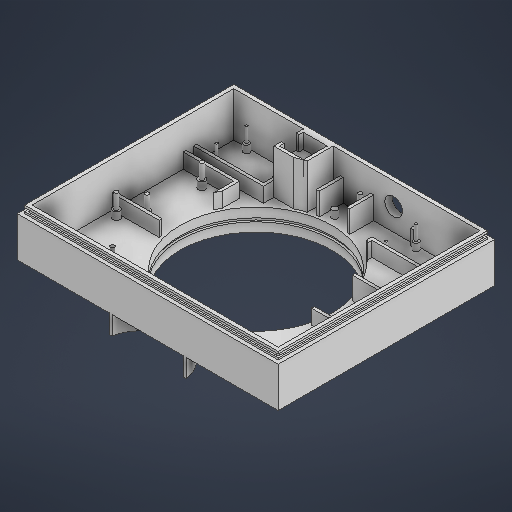
# Autodesk Inventor part: Hardware_Container-bottom-with_rods
Saved by Autodesk Inventor 2026.1 (Build 301233000, 233)
## iProperties
Created: 2025-05-15
Part Number: Hardware_Container-bottom-with_rods
Material: Générique
Document SubType Name: Modeling
Designer: ewenm
Density: 1 g/cm^3
Appearance: Par défaut
Author: ewenm
Autodesk Inventor part; units mm, degrees
ref_plane "YZ Plane" through (0, 0, 0) normal (1, 0, 0) x (0, 1, 0)
ref_plane "XZ Plane" through (0, 0, 0) normal (0, 1, 0) x (-1, 0, 0)
ref_plane "XY Plane" through (0, 0, 0) normal (0, 0, 1) x (1, 0, 0)
sketch "Esquisse1" plane through (0, 0, 0) normal (0, 1, 0) x (-1, 0, 0)
  circle A0 centre (0, 0) radius 51.25
  circle A1 centre (0, 0) radius 53.25
  dimension "d0" = 102.5
  dimension "d1" = 106.5
  constraints: 2 centre point, 2 coincident
  measures "d0" diameter of A0
  measures "d1" diameter of A1
extrude "Extrusion1" add sketch "Esquisse1" along normal blind 12.5
sketch "Esquisse5" plane through (0, 12.5, 0) normal (0, 1, 0) x (1, 0, 0)
  line L0 (-88, -73) -> (88, -73)
  line L1 (88, -73) -> (88, 73)
  line L2 (88, 73) -> (-88, 73)
  line L3 (-88, 73) -> (-88, -73)
  line L4 (-88, -73) -> (88, 73) construction
  line L5 (88, -73) -> (-88, 73) construction
  circle A0 centre (0, 0) radius 51.25
  dimension "d4" = 176
  dimension "d5" = 146
  dimension "d263" = 102.5
  constraints: 12 end point, 2 midpoint, 2 parallel, 1 centre point, 1 coincident, 1 horizontal, 1 perpendicular
  measures "d4" distance of L0.start L0.end
  measures "d5" distance of L1.end L0.end
  measures "d263" diameter of A0
extrude "Extrusion2" add sketch "Esquisse5" along normal blind 2
sketch "Esquisse8" plane through (0, 14.5, 0) normal (0, 1, 0) x (1, 0, 0)
  line L0 (88, -73) -> (88, 73)
  line L1 (88, 73) -> (-88, 73)
  line L2 (-88, 73) -> (-88, -73)
  line L3 (-88, -73) -> (88, -73)
  line L4 (88, -73) -> (-88, 73) construction
  line L5 (88, 73) -> (-88, -73) construction
  line L6 (83, -68) -> (83, 68)
  line L7 (83, 68) -> (-83, 68)
  line L8 (-83, 68) -> (-83, -68)
  line L9 (-83, -68) -> (83, -68)
  line L10 (83, -68) -> (-83, 68) construction
  line L11 (83, 68) -> (-83, -68) construction
  line L12 (88, 73) -> (-88, 73) projected
  point P0 (0, 0)
  dimension "d8" = 136
  dimension "d9" = 166
  dimension "d214" = 146
  dimension "d215" = 176
  dimension "d216" = 0
  constraints: 24 end point, 4 midpoint, 4 parallel, 2 perpendicular, 1 vertical
  measures "d8" distance of L6.start L6.end
  measures "d9" distance of L7.end L6.end
  measures "d214" distance between parallel lines of L1 L3
  measures "d215" distance between parallel lines of L2 L0
  measures "d216" distance between parallel lines of L12 L1
extrude "Extrusion3" add sketch "Esquisse8" along normal blind 25
sketch "Esquisse9" plane through (0, 39.5, 0) normal (0, 1, 0) x (1, 0, 0)
  line L0 (85.5, -70.5) -> (85.5, 70.5)
  line L1 (85.5, 70.5) -> (-85.5, 70.5)
  line L2 (-85.5, 70.5) -> (-85.5, -70.5)
  line L3 (-85.5, -70.5) -> (85.5, -70.5)
  line L4 (85.5, -70.5) -> (-85.5, 70.5) construction
  line L5 (85.5, 70.5) -> (-85.5, -70.5) construction
  line L6 (83, -68) -> (83, 68)
  line L7 (83, 68) -> (-83, 68)
  line L8 (-83, 68) -> (-83, -68)
  line L9 (-83, -68) -> (83, -68)
  line L10 (83, -68) -> (-83, 68) construction
  line L11 (83, 68) -> (-83, -68) construction
  point P0 (0, 0)
  dimension "d12" = 141
  dimension "d13" = 171
  constraints: 24 end point, 4 midpoint, 4 parallel, 2 perpendicular, 1 vertical
  measures "d12" distance of L0.start L0.end
  measures "d13" distance of L1.end L0.end
extrude "Extrusion4" add sketch "Esquisse9" along normal blind 5
sketch "Esquisse10" plane through (0, 14.5, 0) normal (0, 1, 0) x (1, 0, 0)
  line L0 (-83, -68) -> (83, -68) projected
  line L1 (-83, -68) -> (69, -68)
  line L2 (-83, -12.0588) -> (-83, -68)
  line L3 (-83, -68) -> (67, -68)
  line L4 (-83, -14.0686) -> (-83, -68)
  circle A0 centre (0, 0) radius 51.25 projected
  line L5 (69, -12) -> (49.8253, -12)
  line L6 (-49.8111, -12.0588) -> (-83, -12.0588)
  line L7 (67, -14) -> (49.3007, -14)
  line L8 (-49.2812, -14.0686) -> (-83, -14.0686)
  line L9 (67, -43) -> (69, -43)
  line L10 (67, -63) -> (69, -63)
  line L11 (67, -68) -> (67, -63)
  line L12 (67, -43) -> (67, -14)
  line L13 (69, -68) -> (69, -63)
  line L14 (69, -43) -> (69, -12)
  point P0 (51.25, 0)
  point P1 (68, -63)
  point P2 (68, -43)
  dimension "d16" = 152
  dimension "d17" = 56
  dimension "d18" = 150
  dimension "d19" = 54
  dimension "d20" = 5
  dimension "d21" = 20
  constraints: 28 end point, 8 parallel, 8 perpendicular, 5 point on circle, 2 midpoint, 2 point on line, 1 coincident
  measures "d16" distance of L0.start L1.end
  measures "d17" distance of L5.start L1.end
  measures "d18" distance of L0.start L3.end
  measures "d19" distance of L7.start L3.end
  measures "d20" distance from line of L0 point (68, -63)
  measures "d21" distance of point (68, -63) point (68, -43)
extrude "Extrusion5" add sketch "Esquisse10" along normal blind 10 contours L11 L10 L13 L0 | L6 A0 L8 L2 | A0 L5 L14 L9 L12 L7
sketch "Esquisse11" plane through (0, 14.5, 0) normal (0, 1, 0) x (1, 0, 0)
  line L0 (-83, -68) -> (-83, 68) projected
  line L1 (-83, -68) -> (67, -68) projected
  line L2 (-83, 29.4235) -> (-85.5, 61.9088)
  line L3 (-85.5, -70.5) -> (-85.5, 70.5) projected
  line L4 (-83, 33.9412) -> (-49, 33.9412)
  line L5 (-49, 33.9412) -> (-49, 15.0187)
  line L6 (-49.8111, -12.0588) -> (-83, -12.0588) projected
  line L7 (-83, 68) -> (-83, -12.0588) projected
  line L8 (-83, 35.9412) -> (-47, 35.9412)
  line L9 (-47, 35.9412) -> (-47, 20.4343)
  arc A0 (49.8253, -12) -> (-49.8111, -12.0588) centre (0, 0) ccw projected
  arc A1 (-49, 15.0187) -> (-48.1736, 17.489) centre (0, 0) ccw
  point P0 (-83, -20.5374)
  point P1 (-83, 35.9412)
  dimension "d29" = 34
  dimension "d32" = 36
  dimension "d34" = 2
  dimension "d35" = 48
  constraints: 10 end point, 5 point on circle, 5 point on line, 3 perpendicular, 1 centre point, 1 concentric, 1 horizontal
  measures "d29" distance of L4.start L4.end
  measures "d32" distance of L8.start L8.end
  measures "d34" distance between parallel lines of L4 L8
  measures "d35" distance between parallel lines of L8 L6
extrude "Extrusion6" add sketch "Esquisse11" along normal blind 10 contours L0 L8 L9 A0 L5 L4
sketch "Esquisse13" plane through (0, 14.5, 0) normal (0, 1, 0) x (1, 0, 0)
  line L0 (83, 68) -> (-83, 68) projected
  line L1 (-83, 68) -> (-83, 35.9412) projected
  line L2 (-83, 68) -> (-83, 43)
  line L3 (-83, 43) -> (-38, 43)
  line L4 (-38, 43) -> (-38, 68)
  line L5 (-38, 68) -> (-83, 68)
  line L6 (-83, 68) -> (-83, 41)
  line L7 (-83, 41) -> (-36, 41)
  line L8 (-36, 43) -> (-36, 68)
  line L9 (-36, 68) -> (-83, 68)
  line L10 (-36, 68) -> (-36, 43)
  line L11 (13.6206, 68) -> (-36, 68)
  line L12 (-36, 68) -> (-36, 41)
  line L13 (15.4407, 68) -> (-36, 68)
  circle A0 centre (0, 0) radius 51.25 projected
  line L14 (83, 68) -> (38, 68)
  line L15 (83, 43) -> (83, 68)
  line L16 (83, 68) -> (36, 68)
  line L17 (83, 41) -> (83, 68)
  point P0 (-30.4802, 41.201)
  point P1 (-27.557, 43.2108)
  dimension "d49" = 25
  dimension "d50" = 45
  dimension "d51" = 27
  dimension "d52" = 47
  constraints: 32 end point, 4 parallel, 4 point on line, 2 perpendicular, 2 point on circle, 1 collinear
  measures "d49" distance of L0.end L2.end
  measures "d50" distance of L3.end L2.end
  measures "d51" distance of L0.end L6.end
  measures "d52" distance of L7.end L6.end
extrude "Extrusion7" add sketch "Esquisse13" along normal blind 10 contours L8 L12 L7 L1 L3 L4 L0
sketch "Esquisse15" plane through (0, 14.5, 0) normal (0, 1, 0) x (1, 0, 0)
  line L0 (-83, -68) -> (-83, 68) projected
  line L1 (83, -68) -> (-83, -68) projected
  circle A0 centre (-71, -65.05) radius 1.35
  circle A1 centre (-71, -65.05) radius 2.5
  circle A2 centre (-46.9, -49.85) radius 1.35
  circle A3 centre (-46.9, -49.85) radius 2.5
  circle A4 centre (3.9, -65.05) radius 1.35
  circle A5 centre (3.9, -65.05) radius 2.5
  circle A6 centre (-77.32, -16.85) radius 1.35
  circle A7 centre (-77.32, -16.85) radius 2.5
  point P0 (0, 0)
  point P1 (-46.9, -21.95)
  dimension "d63" = 12
  dimension "d64" = 2.95
  dimension "d65" = 15.2
  dimension "d66" = 24.1
  dimension "d67" = 50.8
  dimension "d68" = 0
  dimension "d69" = 2.7
  dimension "d70" = 5
  dimension "d71" = 2.7
  dimension "d72" = 5
  dimension "d73" = 2.7
  dimension "d74" = 5
  dimension "d75" = 27.9
  dimension "d78" = 5.1
  dimension "d79" = 5.68
  dimension "d80" = 2.7
  dimension "d81" = 5
  constraints: 8 centre point, 8 coincident
  measures "d63" distance from line of L0 point (-71, -65.05)
  measures "d64" distance from line of L1 point (-71, -65.05)
  measures "d65" vertical distance of point (-46.9, -49.85) point (-71, -65.05)
  measures "d66" horizontal distance of point (-46.9, -49.85) point (-71, -65.05)
  measures "d67" horizontal distance of point (3.9, -65.05) point (-46.9, -49.85)
  measures "d68" vertical distance of point (-71, -65.05) point (3.9, -65.05)
  measures "d69" diameter of A0
  measures "d70" diameter of A1
  measures "d71" diameter of A2
  measures "d72" diameter of A3
  measures "d73" diameter of A4
  measures "d74" diameter of A5
  measures "d75" distance of A2.centre point (-46.9, -21.95)
  measures "d78" vertical distance of point (-46.9, -21.95) point (-77.32, -16.85)
  measures "d79" distance from line of L0 point (-77.32, -16.85)
  measures "d80" diameter of A6
  measures "d81" diameter of A7
extrude "Extrusion9" add sketch "Esquisse15" along normal blind 5
sketch "Esquisse16" plane through (0, 14.5, 0) normal (0, 1, 0) x (1, 0, 0)
  line L0 (-49, 33.9412) -> (-49, 15.0187) projected
  line L1 (-49.8111, -12.0588) -> (-83, -12.0588) projected
  circle A0 centre (-66, -7.5588) radius 1.35
  circle A1 centre (-66, -7.5588) radius 2.5
  circle A2 centre (-66, 29.4412) radius 1.35
  circle A3 centre (-66, 29.4412) radius 2.5
  point P0 (0, 0)
  dimension "d84" = 17
  dimension "d85" = 17
  dimension "d86" = 37
  dimension "d87" = 4.5
  dimension "d88" = 2.7
  dimension "d89" = 5
  dimension "d90" = 2.7
  dimension "d91" = 5
  constraints: 4 centre point, 4 coincident
  measures "d84" distance from line of L0 point (-66, 29.441)
  measures "d85" distance from line of L0 point (-66, -7.559)
  measures "d86" distance of point (-66, 29.441) point (-66, -7.559)
  measures "d87" distance from line of L1 point (-66, -7.559)
  measures "d88" diameter of A0
  measures "d89" diameter of A1
  measures "d90" diameter of A2
  measures "d91" diameter of A3
sketch "Esquisse17" plane through (0, 14.5, 0) normal (0, 1, 0) x (1, 0, 0)
  line L0 (-38, 43) -> (-38, 68) projected
  line L1 (-38, 68) -> (-83, 68) projected
  line L2 (-83, 43) -> (-38, 43) projected
  circle A0 centre (-42, 55.5) radius 0.85
  circle A1 centre (-42, 55.5) radius 2
  circle A2 centre (-72, 45.4) radius 0.85
  circle A3 centre (-72, 45.4) radius 2
  circle A4 centre (-72, 65.6) radius 0.85
  circle A5 centre (-72, 65.6) radius 2
  line L3 (-83, 68) -> (-83, 43) projected
  line L4 (-42, 55.5) -> (-75.4325, 55.5)
  point P0 (0, 0)
  dimension "d93" = 0
  dimension "d94" = 20.2
  dimension "d95" = 12.5
  dimension "d98" = 1.7
  dimension "d99" = 4
  dimension "d100" = 1.7
  dimension "d101" = 4
  dimension "d102" = 1.7
  dimension "d103" = 4
  dimension "d162" = 11
  dimension "d165" = 30
  dimension "d257" = 10.1
  constraints: 6 centre point, 6 coincident, 2 end point, 1 horizontal
  measures "d93" horizontal distance of point (-72, 45.4) point (-72, 65.6)
  measures "d94" distance of point (-72, 65.6) point (-72, 45.4)
  measures "d95" distance from line of L1 point (-42, 55.5)
  measures "d98" diameter of A0
  measures "d99" diameter of A1
  measures "d100" diameter of A2
  measures "d101" diameter of A3
  measures "d102" diameter of A4
  measures "d103" diameter of A5
  measures "d162" distance from line of L3 point (-72, 65.6)
  measures "d165" horizontal distance of point (-42, 55.5) point (-72, 45.4)
  measures "d257" distance from line of A4.centre L4
extrude "Extrusion10" add sketch "Esquisse16" along normal blind 5
extrude "Extrusion11" add sketch "Esquisse17" along normal blind 5 contours A1 | A3 | A5
sketch "Esquisse18" plane through (-83, 14.5, 68) normal (0, 1, 0) x (1, 0, 0)
  line L0 (166, 136) -> (47, 136) projected
  line L1 (110.9273, 136) -> (135.9273, 136)
  line L2 (166, 136) -> (123, 136)
  line L3 (123, 111) -> (166, 111)
  line L4 (166, 111) -> (166, 136)
  line L5 (166, 136) -> (166, 109)
  line L6 (166, 109) -> (121, 109)
  line L7 (121, 136) -> (166, 136)
  line L8 (123, 113) -> (121, 113)
  line L9 (123, 134) -> (121, 134)
  line L10 (123, 136) -> (123, 134)
  line L11 (123, 113) -> (123, 111)
  line L12 (121, 109) -> (121, 113)
  line L13 (121, 134) -> (121, 136)
  circle A0 centre (125.5, 133.5) radius 0.85
  circle A1 centre (125.5, 133.5) radius 2
  circle A2 centre (125.5, 113.5) radius 0.85
  circle A3 centre (125.5, 113.5) radius 2
  circle A4 centre (163.5, 113.5) radius 0.85
  circle A5 centre (163.5, 113.5) radius 2
  circle A6 centre (163.5, 133.5) radius 0.85
  circle A7 centre (163.5, 133.5) radius 2
  point P0 (83, 68)
  point P1 (122, 113)
  point P2 (122, 134)
  point P3 (123, 135)
  dimension "d109" = 43
  dimension "d110" = 25
  dimension "d111" = 45
  dimension "d112" = 4
  dimension "d113" = 2
  dimension "d114" = 2.5
  dimension "d115" = 2.5
  dimension "d117" = 2.5
  dimension "d118" = 2.5
  dimension "d119" = 2.5
  dimension "d120" = 2.5
  dimension "d121" = 2.5
  dimension "d122" = 2.5
  dimension "d123" = 1.7
  dimension "d124" = 4
  dimension "d125" = 1.7
  dimension "d126" = 4
  dimension "d127" = 1.7
  dimension "d128" = 4
  dimension "d129" = 1.7
  dimension "d130" = 4
  constraints: 26 end point, 10 coincident, 8 centre point, 7 perpendicular, 6 parallel, 3 midpoint, 3 point on line, 1 horizontal
  measures "d109" distance of L3.end L3.start
  measures "d110" distance between parallel lines of L3 L0
  measures "d111" distance of L5.end L6.end
  measures "d112" distance from line of L6 point (122, 113)
  measures "d113" distance from line of L7 point (122, 134)
  measures "d114" distance from line of L5 point (163.5, 133.5)
  measures "d115" distance from line of L7 point (163.5, 133.5)
  measures "d117" horizontal distance of point (123, 135) point (125.5, 133.5)
  measures "d118" distance from line of L7 point (125.5, 133.5)
  measures "d119" distance from line of L11 point (125.5, 113.5)
  measures "d120" distance from line of L3 point (125.5, 113.5)
  measures "d121" distance from line of L3 point (163.5, 113.5)
  measures "d122" distance from line of L4 point (163.5, 113.5)
  measures "d123" diameter of A0
  measures "d124" diameter of A1
  measures "d125" diameter of A2
  measures "d126" diameter of A3
  measures "d127" diameter of A4
  measures "d128" diameter of A5
  measures "d129" diameter of A6
  measures "d130" diameter of A7
extrude "Extrusion12" add sketch "Esquisse18" along normal blind 5 contours A1 | A3 | A5 | A7
sketch "Esquisse19" plane through (-83, 14.5, 68) normal (0, 1, 0) x (1, 0, 0)
  line L0 (166, 0) -> (166, 136) projected
  line L1 (166, 136) -> (166, 111)
  line L2 (166, 111) -> (123, 111)
  line L3 (123, 136) -> (166, 136)
  line L4 (166, 136) -> (166, 109)
  line L5 (166, 109) -> (121, 109)
  line L6 (121, 136) -> (166, 136)
  line L7 (123, 113) -> (121, 113)
  line L8 (123, 134) -> (121, 134)
  line L9 (123, 111) -> (123, 113)
  line L10 (123, 134) -> (123, 136)
  line L11 (121, 109) -> (121, 113)
  line L12 (121, 134) -> (121, 136)
  point P0 (83, 68)
  point P1 (122, 134)
  point P2 (122, 113)
  dimension "d133" = 43
  dimension "d134" = 45
  dimension "d135" = 2
  dimension "d136" = 2
  constraints: 24 end point, 6 parallel, 6 perpendicular, 2 midpoint, 2 point on line
  measures "d133" distance of L1.end L2.end
  measures "d134" distance of L4.end L5.end
  measures "d135" distance from line of L6 point (122, 134)
  measures "d136" distance from line of L2 point (122, 113)
extrude "Extrusion13" add sketch "Esquisse19" along normal blind 10
sketch "Esquisse22" plane through (-83, 44.5, -68) normal (0, 0, 1) x (1, 0, 0)
  line L0 (121, -30) -> (123, -30) projected
  line L1 (94.8124, -20) -> (94.8124, -30) projected
  point P0 (83, -44.5)
  point P1 (107.8124, -15)
  point P2 (122, -30)
  dimension "d153" = 15
  dimension "d154" = 13
  constraints: 1 midpoint
  measures "d153" vertical distance of point (122, -30) point (107.812, -15)
  measures "d154" distance from line of point (107.812, -15) L1
hole "Perçage2" at (24.8124, 29.5, -68) direction (0, 0, -1) diameter 12 end through all
sketch "Esquisse24" plane through (0, 14.5, 0) normal (0, 1, 0) x (1, 0, 0)
  line L0 (-36, 68) -> (-36, 41) projected
  line L1 (-36, 68) -> (-16, 68)
  line L2 (-16, 68) -> (-16, 48)
  line L3 (-16, 48) -> (-36, 48)
  line L4 (-36, 48) -> (-36, 68)
  point P0 (0, 0)
  dimension "d166" = 20
  dimension "d167" = 20
  constraints: 8 end point, 2 parallel, 1 horizontal, 1 perpendicular
  measures "d166" distance of L2.end L3.end
  measures "d167" distance of L1.end L2.end
extrude "Extrusion15" add sketch "Esquisse24" along normal blind 20
sketch "Esquisse26" plane through (0, 34.5, 0) normal (0, 1, 0) x (1, 0, 0)
  line L0 (-36, 48) -> (-36, 68) projected
  line L1 (-36, 48) -> (-16, 48) projected
  line L2 (-36, 68) -> (-16, 68)
  line L3 (-16, 68) -> (-16, 48)
  line L4 (-16, 48) -> (-36, 48)
  line L5 (-34, 66) -> (-18, 66)
  line L6 (-18, 66) -> (-18, 50)
  line L7 (-18, 50) -> (-34, 50)
  line L8 (-34, 63) -> (-36, 63)
  line L9 (-34, 53) -> (-36, 53)
  line L10 (-34, 50) -> (-34, 53)
  line L11 (-34, 63) -> (-34, 66)
  line L12 (-36, 48) -> (-36, 53)
  line L13 (-36, 63) -> (-36, 68)
  point P0 (0, 0)
  point P1 (-26, 66)
  point P2 (-35, 53)
  point P3 (-35, 63)
  point P4 (-34, 68)
  point P5 (-34, 65)
  point P6 (-34, 65)
  dimension "d174" = 16
  dimension "d175" = 16
  dimension "d177" = 2
  dimension "d178" = 3
  dimension "d179" = 3
  dimension "d258" = 2
  dimension "d259" = 0
  dimension "d260" = 2
  constraints: 24 end point, 6 parallel, 5 perpendicular, 3 midpoint, 2 horizontal
  measures "d174" distance of L6.end L7.end
  measures "d175" distance of L5.end L6.end
  measures "d177" distance from line of L2 point (-26, 66)
  measures "d178" distance from line of L7 point (-35, 53)
  measures "d179" distance from line of L5 point (-35, 63)
  measures "d258" distance between parallel lines of L3 L6
  measures "d259" distance between parallel lines of L0 L12
  measures "d260" distance between parallel lines of L0 L11
extrude "Extrusion16" add sketch "Esquisse26" along normal blind 10 contours L0 L9 L10 L7 L6 L5 L11 L8 L2 L3 L1
sketch "Esquisse27" plane through (0, 14.5, 0) normal (0, 1, 0) x (1, 0, 0)
  line L0 (38, 41) -> (83, 41) projected
  line L1 (83, 41) -> (37.1814, 41)
  line L2 (37.1814, 41) -> (37.1814, 35.2719)
  line L3 (48.6626, 16.0784) -> (83, 16.0784)
  line L4 (83, 16.0784) -> (83, 41)
  line L5 (83, 43) -> (83, 68) projected
  line L6 (83, 43) -> (35.1716, 43)
  line L7 (35.1716, 43) -> (35.1716, 37.2763)
  line L8 (49.2812, 14.0686) -> (83, 14.0686)
  line L9 (83, 14.0686) -> (83, 43)
  arc A0 (-49, 15.0187) -> (-49.8111, -12.0588) centre (0, 0) ccw projected
  circle A1 centre (0, 0) radius 51.25 projected
  arc A2 (49.2812, 14.0686) -> (48.6626, 16.0784) centre (0, 0) ccw
  arc A3 (37.1814, 35.2719) -> (35.1716, 37.2763) centre (0.1766, 0.1771) ccw
  point P0 (-47, 20.4343)
  point P1 (49.8253, -12)
  point P2 (48.4252, 16)
  point P3 (49.0408, 14)
  constraints: 16 end point, 10 point on circle, 4 parallel, 2 centre point, 2 horizontal, 2 perpendicular, 1 concentric
extrude "Extrusion17" add sketch "Esquisse27" along normal blind 15 contours L1 L2 A1 L7 L6 L9 L0 | L9 L8 A1 L3
sketch "Esquisse28" plane through (0, 14.5, 0) normal (0, 1, 0) x (1, 0, 0)
  line L0 (38, 68) -> (-16, 68) projected
  line L1 (-9.25, 68) -> (9.25, 68)
  line L2 (9.25, 68) -> (9.25, 50.4083)
  line L3 (-9.25, 50.4083) -> (-9.25, 68)
  line L4 (-11.25, 68) -> (11.25, 68)
  line L5 (11.25, 68) -> (11.25, 50)
  line L6 (-11.25, 50) -> (-11.25, 68)
  circle A0 centre (5.75, 64.5) radius 1.35
  circle A1 centre (5.75, 64.5) radius 2
  arc A2 (-49, 15.0187) -> (-49.8111, -12.0588) centre (0, 0) ccw projected
  arc A3 (-9.25, 50.4083) -> (-11.25, 50) centre (-0.05, 0.245) ccw
  arc A4 (11.25, 50) -> (9.25, 50.4083) centre (0, 0) ccw
  line L7 (0, 0) -> (0, 99.0473)
  circle A5 centre (-3.9912, 57.0747) radius 2
  line L8 (-83, -68) -> (-83, 68) projected
  point P0 (-47, 20.4343)
  point P1 (35, 37.0945)
  dimension "d194" = 3.5
  dimension "d195" = 3.5
  dimension "d200" = 2.7
  dimension "d201" = 4
  dimension "d236" = 18.5
  dimension "d237" = 4
  dimension "d238" = 83
  dimension "d239" = 2
  dimension "d240" = 2
  constraints: 14 end point, 8 point on circle, 5 centre point, 2 coincident, 2 horizontal, 2 parallel, 2 perpendicular, 2 point on line, 1 vertical, 1 other
  measures "d194" distance from line of L0 point (5.75, 64.5)
  measures "d195" distance from line of L2 point (5.75, 64.5)
  measures "d200" diameter of A0
  measures "d201" diameter of A1
  measures "d236" distance between parallel lines of L2 L3
  measures "d237" diameter of A5
  measures "d238" distance between parallel lines of L8 L7
  measures "d239" distance between parallel lines of L3 L6
  measures "d240" distance between parallel lines of L5 L2
extrude "Extrusion18" add sketch "Esquisse28" along normal blind 5
sketch "Esquisse30" plane through (0, 19.5, 0) normal (0, 1, 0) x (1, 0, 0)
  line L0 (-9.25, 50.01) -> (-9.25, 68)
  line L1 (-9.25, 68) -> (-11.25, 68)
  line L2 (-11.25, 68) -> (-11.25, 49.7437)
  arc A0 (11.25, 50) -> (9.25, 50.4083) centre (0, 0) ccw projected
  line L3 (9.25, 68) -> (9.25, 50.4083) projected
  line L4 (9.25, 50.4083) -> (9.25, 68)
  line L5 (9.25, 68) -> (11.25, 68)
  line L6 (11.25, 68) -> (11.25, 50)
  arc A1 (-9.25, 50.01) -> (-11.25, 49.7437) centre (-3.5206, -0.6671) ccw
  arc A2 (11.25, 50) -> (9.25, 50.4083) centre (0.05, 0.245) ccw
  constraints: 12 end point, 5 point on circle, 2 centre point, 2 parallel, 1 collinear, 2 other
extrude "Extrusion19" add sketch "Esquisse30" along normal blind 10
sketch "Esquisse32" plane through (0, 0, 0) normal (0, -1, 0) x (1, 0, 0)
  circle A0 centre (0, 0) radius 51.5
  circle A1 centre (0, 0) radius 52.75
  dimension "d209" = 105.5
  dimension "d210" = 103
  constraints: 2 centre point, 2 coincident
  measures "d209" diameter of A1
  measures "d210" diameter of A0
ref_plane "Plan de construction1" through (0, 6, 0) normal (0, -1, 0) x (1, 0, 0)
extrude "Extrusion21" cut sketch "Esquisse32" against normal blind 2.3 from surface at -6 contours A0 | A1
sketch "Esquisse33" plane through (0, 44.5, 0) normal (0, 1, 0) x (1, 0, 0)
  line L0 (-85.5, -70.5) -> (-85.5, 70.5) projected
  line L1 (85.5, -70.5) -> (85.5, 70.5) projected
  line L2 (-85.5, -70.5) -> (85.5, -70.5)
  line L3 (85.5, -70.5) -> (85.5, 70.5)
  line L4 (85.5, 70.5) -> (-85.5, 70.5)
  line L5 (-85.5, 70.5) -> (-85.5, -70.5)
  line L6 (-84.5, -69.5) -> (84.5, -69.5)
  line L7 (84.5, -69.5) -> (84.5, 69.5)
  line L8 (84.5, 69.5) -> (-84.5, 69.5)
  line L9 (-84.5, 69.5) -> (-84.5, -69.5)
  point P0 (0, 0)
  point P1 (85.5, -70.5)
  point P2 (-85.5, 70.5)
  dimension "d217" = 1
  dimension "d218" = 1
  dimension "d219" = 1
  dimension "d220" = 1
  constraints: 16 end point, 4 parallel, 2 horizontal, 2 perpendicular
  measures "d217" distance between parallel lines of L0 L9
  measures "d218" distance between parallel lines of L4 L8
  measures "d219" distance between parallel lines of L2 L6
  measures "d220" distance between parallel lines of L1 L7
ref_plane "Plan de construction2" through (0, 43, 0) normal (0, 1, 0) x (1, 0, 0)
extrude "Extrusion22" cut sketch "Esquisse33" against normal blind 2.3 from surface at -1.5
sketch "Esquisse35" plane through (0, 14.5, 0) normal (0, 1, 0) x (1, 0, 0)
  circle A0 centre (0, 0) radius 53
  dimension "d230" = 106
  constraints: 1 centre point, 1 coincident
  measures "d230" diameter of A0
sketch "Esquisse36" plane through (0, 14.5, 0) normal (0, 1, 0) x (1, 0, 0)
  line L0 (83, 41) -> (37.1814, 41) projected
  line L1 (83, 16.0784) -> (48.6626, 16.0784) projected
  line L2 (37.1814, 41) -> (83, 41)
  line L3 (83, 41) -> (83, 16.0784)
  line L4 (83, 16.0784) -> (37.1814, 16.0784)
  line L5 (37.1814, 16.0784) -> (37.1814, 41)
  point P0 (0, 0)
  point P1 (50.5272, 16)
  point P2 (50.5272, 16)
  point P3 (48.4252, 16)
  constraints: 6 end point, 2 horizontal, 1 parallel, 1 perpendicular, 4 other
extrude "Extrusion26" add sketch "Esquisse36" along normal blind 5
extrude "Extrusion27" cut sketch "Esquisse35" along normal up to surface (30 mm away)
sketch "Esquisse37" plane through (0, 12.5, 0) normal (0, -1, 0) x (1, 0, 0)
  circle A0 centre (0, 0) radius 53
  line L0 (-88, 73) -> (88, 73) projected
  line L1 (-24.5, 73) -> (-24.5, 46.9973)
  line L2 (24.5, 73) -> (24.5, 46.9973)
  line L3 (26.5, 73) -> (26.5, 45.8993)
  line L4 (-26.5, 73) -> (-26.5, 45.8993)
  line L5 (-19.7568, 53) -> (19.0821, 53)
  circle A1 centre (0, 0) radius 51.25 projected
  line L6 (-21.3391, 51) -> (19.9361, 51)
  circle A2 centre (0, 77.5) radius 24.5
  circle A3 centre (0, 77.5) radius 26.5
  line L7 (-26.1151, 73) -> (-24.0832, 73)
  line L8 (24.0832, 73) -> (26.1151, 73)
  point P0 (-24.5, 59.9987)
  point P1 (0, 53)
  point P2 (8.326, 52.3419)
  point P3 (-8.326, 52.3419)
  point P4 (49.3007, 14)
  point P5 (-49.2812, 14.0686)
  point P6 (0, 73)
  point P7 (0, 73)
  dimension "d247" = 24.5
  dimension "d248" = 106
  dimension "d249" = 24.5
  dimension "d250" = 2
  dimension "d251" = 2
  dimension "d267" = 77.5
  dimension "d268" = 4.5
  constraints: 16 end point, 8 point on circle, 6 tangent, 3 centre point, 3 parallel, 2 coincident, 1 horizontal, 1 midpoint, 1 vertical, 10 other
  measures "d247" horizontal distance of point (0, 0) point (-24.5, 59.999)
  measures "d248" diameter of A0
  measures "d249" distance from line of point (0, 0) L2
  measures "d250" distance between parallel lines of L3 L2
  measures "d251" distance between parallel lines of L1 L4
  measures "d267" distance of point (0, 0) A2.centre
  measures "d268" distance of point (0, 73) point (0, 77.5)
sketch "Esquisse38" plane through (0, 14.5, 0) normal (0, 1, 0) x (1, 0, 0)
  circle A0 centre (-46.9, -49.85) radius 1.35 projected
  circle A1 centre (-46.9, -49.85) radius 1.35
  circle A2 centre (-71, -65.05) radius 1.35 projected
  circle A3 centre (-71, -65.05) radius 1.35
  circle A4 centre (3.9, -65.05) radius 1.35 projected
  circle A5 centre (3.9, -65.05) radius 1.35
  circle A6 centre (-77.32, -16.85) radius 1.35 projected
  circle A7 centre (-77.32, -16.85) radius 1.35
  circle A8 centre (-66, -7.5588) radius 1.35 projected
  circle A9 centre (-66, -7.5588) radius 1.35
  circle A10 centre (-66, 29.4412) radius 1.35 projected
  circle A11 centre (-66, 29.4412) radius 1.35
  circle A12 centre (-72, 45.4) radius 0.85 projected
  circle A13 centre (-72, 45.4) radius 0.85
  circle A14 centre (-72, 65.6) radius 0.85 projected
  circle A15 centre (-72, 65.6) radius 0.85
  circle A16 centre (-42, 55.5) radius 0.85 projected
  circle A17 centre (-42, 55.5) radius 0.85
  circle A18 centre (5.75, 64.5) radius 1.35 projected
  circle A19 centre (5.75, 64.5) radius 1.35
  circle A20 centre (42.5, 45.5) radius 0.85 projected
  circle A21 centre (42.5, 45.5) radius 0.85
  circle A22 centre (42.5, 65.5) radius 0.85 projected
  circle A23 centre (42.5, 65.5) radius 0.85
  circle A24 centre (80.5, 65.5) radius 0.85 projected
  circle A25 centre (80.5, 65.5) radius 0.85
  circle A26 centre (80.5, 45.5) radius 0.85 projected
  circle A27 centre (80.5, 45.5) radius 0.85
  point P0 (0, 0)
  constraints: 14 centre point, 14 coincident
extrude "Extrusion30" add sketch "Esquisse38" along normal blind 15
extrude "Extrusion32" add sketch "Esquisse37" along normal blind 12.5 contours A3 L5 A2 L0 L2 | L2 L0 A3 | A3 L0 L1 | L1 L0 A2 L5 A3 | A0 L5 A3 | A3 L5 A0
fillet "Congé2" radius 1 4 edges at (84.5, 41.85, -69.5) (84.5, 41.85, 69.5) (-84.5, 41.85, 69.5) (-84.5, 41.85, -69.5)
equation "\"d168\" = d166"
